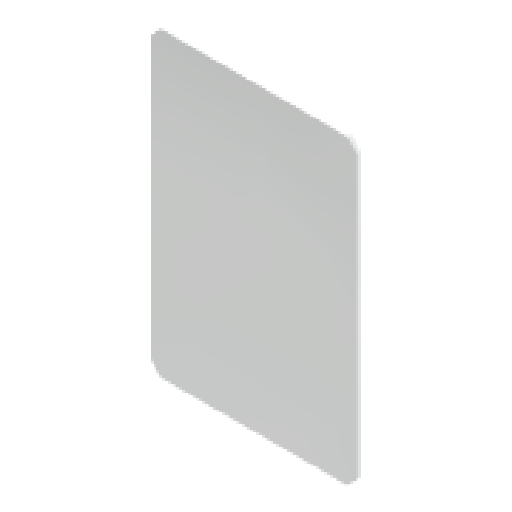
# Autodesk Inventor part: Heated Bed Glass
Saved by Autodesk Inventor 2023.2 (Build 272271000, 271)
## iProperties
Created: 2023-02-02
Part Number: Heated Bed Glass
Material: Glass
Document SubType Name: Modeling
Designer: remop
Density: 2.18 g/cm^3
Appearance: Clear
Author: remop
Autodesk Inventor part; units mm, degrees
ref_plane "YZ Plane" through (0, 0, 0) normal (1, 0, 0) x (0, 1, 0)
ref_plane "XZ Plane" through (0, 0, 0) normal (0, 1, 0) x (-1, 0, 0)
ref_plane "XY Plane" through (0, 0, 0) normal (0, 0, 1) x (1, 0, 0)
sketch "Sketch1" plane through (0, 0, 0) normal (0, 0, 1) x (1, 0, 0)
  line L0 (107, -157) -> (-107, -157)
  line L1 (-107, -157) -> (-107, 157)
  line L2 (-107, 157) -> (107, 157)
  line L3 (107, 157) -> (107, -157)
  line L4 (107, -157) -> (-107, 157) construction
  line L5 (-107, -157) -> (107, 157) construction
  point P0 (0, 0)
  dimension "d0" = 314
  dimension "d1" = 214
  constraints: 12 end point, 2 midpoint, 2 parallel, 1 horizontal, 1 perpendicular
  measures "d0" distance of L0.end L1.end
  measures "d1" distance of L1.end L2.end
extrude "Extrusion1" add sketch "Sketch1" along normal blind 4
chamfer "Chamfer1" distance 10.5 angle 45 4 edges at (-107, 157, 2) (-107, -157, 2) (107, -157, 2) (107, 157, 2)
body "Solid1"
